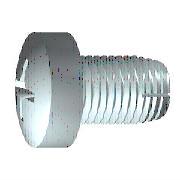
# Autodesk Inventor part: ANSI B18.6.4 - No. 4 - 40 - 1/4, CRFHTSTDTI(2)
Saved by Autodesk Inventor 2026.1 (Build 301233000, 233)
## iProperties
Created: 2025-01-21
Part Number: ANSI B18.6.4 - No. 4 - 40 - 1/4, CRFHTSTDTI(2)
Material: Steel, Mild
Description: Cross Recessed Fillister Head Tapping Screw - Type D - Type I
Document SubType Name: Modeling
Standard: ANSI B18.6.4
Designer: momen
Standard Revision: 1998
Standards Organization: ANSI
Language: en-US
Size Designation: No. 4 - 40 - 1/4
Categories: <MemberInstance><Categories><Category DisplayName="Fasteners" InternalName="e4da775c-781d-43d5-af7c-5136215cf5a6" Mnemonic="FSTN"><Category DisplayName="Bolts" InternalName="536e6df0-f778-49ac-b2f2-25c71d2aa0b2" Mnemonic="SCRW"><CategoryParameter DisplayName="Nominal Diameter Designation" InternalName="03caf894-eafd-4c09-a035-916ac084b87b" Mnemonic="nomdiadesig"/><CategoryParameter DisplayName="Nominal Length" InternalName="238ecbaf-3e6c-45dd-aa95-4068c8e0fd02" Mnemonic="nomlen"/><CategoryParameter DisplayName="Thread Designation" InternalName="586d5e89-370a-4089-914f-0110033585c7" Mnemonic="thrdesign"/><CategoryParameter DisplayName="Thread Series Designation" InternalName="87c5849c-b3a5-4c3e-9c9b-2feecef9be86" Mnemonic="thrserdsgn"/><CategoryParameter DisplayName="Nominal Diameter" InternalName="8bbe3f8e-44cf-40a9-a251-3a6edc8168d6" Mnemonic="nomdia"/><CategoryParameter DisplayName="Thread Type" InternalName="b4bbb7bc-d6aa-4c9f-a9a9-4152b9f6fe49" Mnemonic="thrtype"/><CategoryParameter DisplayName="Thread Pitch" InternalName="bb82302e-82d8-4176-8fc1-c5d7bb17d5ad" Mnemonic="pitch1"/><CategoryParameter DisplayName="Threads per Unit" InternalName="bdc6e7d2-ffd0-4d9c-a173-16b95ebb912d" Mnemonic="thrperunit1"/><CategoryParameter DisplayName="Thread Class" InternalName="ebc0d23b-2cc6-4d2a-b376-d52aae53bab6" Mnemonic="thrclss"/><Category DisplayName="Round Head" InternalName="df3578aa-538f-4805-96a8-2439eb0c3cf7" Mnemonic="RNDSCRW"><CategoryParameter DisplayName="Grip Length" InternalName="2c6ace26-543b-4217-91c4-9cdf8c3ec6f1" Mnemonic="grplen"/><CategoryParameter DisplayName="Head Height" InternalName="2d152238-84fe-49ae-94c3-3fee884c292b" Mnemonic="headh"/><CategoryParameter DisplayName="Property Class" InternalName="85496db6-1567-48ed-b0d4-aa1f03366005" Mnemonic="propclss"/><CategoryParameter DisplayName="Thread Length" InternalName="a1e5edc5-4ca7-4847-8786-65b14d35af16" Mnemonic="thrlen"/><CategoryParameter DisplayName="Shank Diameter" InternalName="c22f1a48-b8d5-43ef-ac5e-546ba91c0bd6" Mnemonic="grpdia"/><CategoryParameter DisplayName="Head Diameter" InternalName="e71ee7a1-06fd-425c-ba3b-09769885677c" Mnemonic="headdia"/><Category DisplayName="Self Tapping Screws" InternalName="33fb404f-0d7c-4133-a804-5105a5fcc9da" Mnemonic="RNDCNRGTPSCRW"/></Category></Category></Category><Category DisplayName="DataType" InternalName="23b78d0f-2648-40c6-8793-ca6db495c9e8" Mnemonic="DATATYPE"><CategoryParameter DisplayName="DisplayName" InternalName="05415f3d-3907-474b-a020-eb9d644f4cf3" Mnemonic="DISPLAYNAME"/><CategoryParameter DisplayName="Standard" InternalName="0c0a119c-1e12-4c84-803f-101930972f5e" Mnemonic="STANDARD"/><CategoryParameter DisplayName="Description" InternalName="13903e3d-64b1-4950-80da-f627842ea37f" Mnemonic="DESCRIPTION"/><CategoryParameter DisplayName="Designation" InternalName="2675968c-4ce5-49e0-a4f5-552d29089031" Mnemonic="DESIGNATION"/><CategoryParameter DisplayName="Default Row" InternalName="2af9ec52-faaa-4026-b378-f9fa4afca842" Mnemonic="DEFAULTROW"/><CategoryParameter DisplayName="Folder Name" InternalName="3f06958e-8713-4116-9be7-ed6184ecc97b" Mnemonic="FOLDERNAME"/><CategoryParameter DisplayName="Revision Guid" InternalName="45a75005-10b1-4dfc-8d6d-dfe629f0b93c" Mnemonic="REVISIONGUID"/><CategoryParameter DisplayName="FileName" InternalName="8b46a4cc-9585-4fed-90c3-899f57e09a73" Mnemonic="FILENAME"/><CategoryParameter DisplayName="StdsOrg" InternalName="8f5914e1-4693-403f-8ab5-d37768198c9d" Mnemonic="STDSORG"/><CategoryParameter DisplayName="Family Version" InternalName="914462f6-6e19-4b14-ba84-155b9680b1d0" Mnemonic="FAMILYREVISION"/><CategoryParameter DisplayName="Standard Revision" InternalName="91d5a463-65c2-4fde-b823-3b7fea5e8e17" Mnemonic="STANDARDREVISION"/><CategoryParameter DisplayName="Member Revision" InternalName="a65d44b9-392f-4f4f-857b-e4b3d54996fe" Mnemonic="MEMBERREVISION"/><CategoryParameter DisplayName="ClipFormat" InternalName="bc51e27b-3422-4e78-93ef-cec197ddf230" Mnemonic="CLIPFORMAT"/><CategoryParameter DisplayName="Manufacturer" InternalName="cd6c7a72-a28a-4e50-99a9-2c7f4e13e5ad" Mnemonic="MANUFACTURER"/><CategoryParameter DisplayName="InternalName" InternalName="cf1d0246-76d9-4b4a-8305-fa0409afb5c1" Mnemonic="INTERNALNAME"/><CategoryParameter DisplayName="IsMetric" InternalName="e2385c5b-1ea4-4823-96a8-8de651266ec3" Mnemonic="ISMETRIC"/><Category DisplayName="Part" InternalName="c0e0b642-3bcb-4cc8-9e80-f96d35c4afa4" Mnemonic="PART"><CategoryParameter DisplayName="Part Number" InternalName="016b6077-bfbe-49bd-92c9-d8d59c39c941" Mnemonic="PARTNUMBER"/><CategoryParameter DisplayName="Stock Number" InternalName="4dba7c1c-e26c-444e-836c-b08b433409a8" Mnemonic="STOCKNUMBER"/><CategoryParameter DisplayName="Material Key" InternalName="5c9a8adb-dd2b-4535-b97f-0a94a95fe41f" Mnemonic="MATERIALKEY"/><CategoryParameter DisplayName="Material" InternalName="818a152a-d3c3-49ca-80ee-df7d91421b8e" Mnemonic="MATERIAL"/></Category></Category><Category DisplayName="LegacyMap" InternalName="cd87c42b-3e48-431e-b5c0-1cbeb14dfe77" Mnemonic="LEGACYMAP"><CategoryParameter DisplayName="unique DA member ID" InternalName="0918ad47-427f-4fed-ae26-24c81c58f590" Mnemonic="DACOOKIE"/><CategoryParameter DisplayName="Merge11 ID" InternalName="0ee8fb18-e2ed-4f39-96f6-1f4b5f50aa71" Mnemonic="MERGE11"/><CategoryParameter DisplayName="unique CC member ID" InternalName="5193edd4-b2b0-4ab4-9d54-de900eee34e0" Mnemonic="CCCOOKIE"/><CategoryParameter DisplayName="Split ID" InternalName="72b5c83c-be7f-45c4-ae51-9160ea6deb26" Mnemonic="SPLIT"/><CategoryParameter DisplayName="MemberID" InternalName="8e5e0294-fc51-4c8f-b3d7-003dc5ed94f6" Mnemonic="MEMBERID"/><CategoryParameter DisplayName="CatalogName" InternalName="d99d1e27-aa94-4de2-af4c-c348882a6f4f" Mnemonic="CATALOGNAME"/><CategoryParameter DisplayName="FamilyNumber" InternalName="e705e1f4-09cb-413e-91f9-551b4188271e" Mnemonic="FAMILYNUMBER"/></Category></Categories><FamilyTemplate Id="sa0009"><FamilyTemplateParameters><FamilyTemplateParameter ObjectType="kUserParameterObject" ValueType="xs:double" Id="1" ObjectReferenceKey="KOH"/><FamilyTemplateParameter ObjectType="kUserParameterObject" ValueType="xs:double" Id="2" ObjectReferenceKey="GD2"/><FamilyTemplateParameter ObjectType="kUserParameterObject" ValueType="xs:double" Id="3" ObjectReferenceKey="KOD"/><FamilyTemplateParameter ObjectType="kUserParameterObject" ValueType="xs:double" Id="4" ObjectReferenceKey="SBR"/><FamilyTemplateParameter ObjectType="kUserParameterObject" ValueType="xs:double" Id="5" ObjectReferenceKey="KR"/><FamilyTemplateParameter ObjectType="kUserParameterObject" ValueType="xs:double" Id="6" ObjectReferenceKey="GEL"/><FamilyTemplateParameter ObjectType="kUserParameterObject" ValueType="xs:double" Id="7" ObjectReferenceKey="THREADDIA"/><FamilyTemplateParameter ObjectType="kUserParameterObject" ValueType="xs:double" Id="8" ObjectReferenceKey="TOA"/><FamilyTemplateParameter ObjectType="kUserParameterObject" ValueType="xs:double" Id="9" ObjectReferenceKey="NLG"/><FamilyTemplateParameter ObjectType="kUserParameterObject" ValueType="xs:double" Id="10" ObjectReferenceKey="STI"/><FamilyTemplateParameter ObjectType="kUserParameterObject" ValueType="xs:double" Id="11" ObjectReferenceKey="TPU"/><FamilyTemplateParameter ObjectType="kUserParameterObject" ValueType="xs:double" Id="12" ObjectReferenceKey="PTC"/><FamilyTemplateParameter ObjectType="kUserParameterObject" ValueType="xs:double" Id="13" ObjectReferenceKey="SDM"/><FamilyTemplateParameter ObjectType="kUserParameterObject" ValueType="xs:double" Id="14" ObjectReferenceKey="NND"/><FamilyTemplateParameter ObjectType="kUserParameterObject" ValueType="xs:double" Id="15" ObjectReferenceKey="SPTZ"/><FamilyTemplateParameter ObjectType="kUserParameterObject" ValueType="xs:double" Id="16" ObjectReferenceKey="GD1"/><FamilyTemplateParameter ObjectType="kPropertyObject" ValueType="xs:string" Id="100" ObjectReferenceKey="{32853F0F-3444-11d1-9E93-0060B03C1CA6}" SubObjectId="52"/><FamilyTemplateParameter ObjectType="kPropertyObject" ValueType="xs:string" Id="105" ObjectReferenceKey="{32853F0F-3444-11d1-9E93-0060B03C1CA6}" SubObjectId="5"/><FamilyTemplateParameter ObjectType="kPartComponentDefinitionObject" ValueType="xs:string" Id="110" SubObjectId="Material"/><FamilyTemplateParameter ObjectType="kThreadFeatureObject" ValueType="xs:structure" Id="300" ObjectReferenceKey="1002000010000000f2360000000000008000000000000000" SubObjectId="ThreadInfo"><FamilyTemplateParameter ObjectType="" ValueType="xs:string" Id="301" SubObjectId="ThreadDesignation"/><FamilyTemplateParameter ObjectType="" ValueType="xs:string" Id="302" SubObjectId="ThreadClass"/><FamilyTemplateParameter ObjectType="" ValueType="xs:string" Id="303" SubObjectId="ThreadType"/></FamilyTemplateParameter></FamilyTemplateParameters></FamilyTemplate><CategoryParameterMap><ParamToTemplateMap><ParamToTemplate CategoryParameter="//CategoryParameter[@InternalName='05415f3d-3907-474b-a020-eb9d644f4cf3']" ConstantValue="Cross Recessed Fillister Head Tapping Screw - Type D - Type I"/><ParamToTemplate CategoryParameter="//CategoryParameter[@InternalName='cf1d0246-76d9-4b4a-8305-fa0409afb5c1']" ConstantValue="8080ad6c-c1cb-4074-8ae5-e7158f342324"/><ParamToTemplate CategoryParameter="//CategoryParameter[@InternalName='3f06958e-8713-4116-9be7-ed6184ecc97b']" ConstantValue="ANSI B18.6.4(33)"/><ParamToTemplate CategoryParameter="//CategoryParameter[@InternalName='914462f6-6e19-4b14-ba84-155b9680b1d0']" ConstantValue="10"/><ParamToTemplate CategoryParameter="//CategoryParameter[@InternalName='bc51e27b-3422-4e78-93ef-cec197ddf230']" ConstantValue="CF_INVENTOR.STDPARTS"/><ParamToTemplate CategoryParameter="//CategoryParameter[@InternalName='e2385c5b-1ea4-4823-96a8-8de651266ec3']" ConstantValue="false"/><ParamToTemplate CategoryParameter="//CategoryParameter[@InternalName='13903e3d-64b1-4950-80da-f627842ea37f']" ConstantValue="Cross Recessed Fillister Head Tapping Screw - Type D - Type I"/><ParamToTemplate CategoryParameter="//CategoryParameter[@InternalName='8f5914e1-4693-403f-8ab5-d37768198c9d']" ConstantValue="ANSI"/><ParamToTemplate CategoryParameter="//CategoryParameter[@InternalName='0c0a119c-1e12-4c84-803f-101930972f5e']" ConstantValue="ANSI B18.6.4"/><ParamToTemplate CategoryParameter="//CategoryParameter[@InternalName='cd6c7a72-a28a-4e50-99a9-2c7f4e13e5ad']" TemplateParameter="104"/><ParamToTemplate CategoryParameter="//CategoryParameter[@InternalName='91d5a463-65c2-4fde-b823-3b7fea5e8e17']" ConstantValue="1998"/><ParamToTemplate CategoryParameter="//CategoryParameter[@InternalName='45a75005-10b1-4dfc-8d6d-dfe629f0b93c']" ConstantValue="b6542b49-97e1-4268-8fde-ea025e42451f"/><ParamToTemplate CategoryParameter="//CategoryParameter[@InternalName='2af9ec52-faaa-4026-b378-f9fa4afca842']" ConstantValue="10"/><ParamToTemplate CategoryParameter="//CategoryParameter[@InternalName='d99d1e27-aa94-4de2-af4c-c348882a6f4f']" ConstantValue="ANSI"/><ParamToTemplate CategoryParameter="//CategoryParameter[@InternalName='e705e1f4-09cb-413e-91f9-551b4188271e']" ConstantValue="949"/><ParamToTemplate CategoryParameter="//CategoryParameter[@InternalName='8b46a4cc-9585-4fed-90c3-899f57e09a73']" ConstantValue="ANSI B18.6.4 - 4-40 UNC - 0.25(3) D I"/><ParamToTemplate CategoryParameter="//CategoryParameter[@InternalName='a65d44b9-392f-4f4f-857b-e4b3d54996fe']" ConstantValue="A9A2BEB8-BFFA-4478-AFC5-B98419E7CDA5"/><ParamToTemplate CategoryParameter="//CategoryParameter[@InternalName='c22f1a48-b8d5-43ef-ac5e-546ba91c0bd6']" ConstantValue="0.112"/><ParamToTemplate CategoryParameter="//CategoryParameter[@InternalName='2c6ace26-543b-4217-91c4-9cdf8c3ec6f1']" ConstantValue="0"/><ParamToTemplate CategoryParameter="//CategoryParameter[@InternalName='ebc0d23b-2cc6-4d2a-b376-d52aae53bab6']" ConstantValue="2A"/><ParamToTemplate CategoryParameter="//CategoryParameter[@InternalName='b4bbb7bc-d6aa-4c9f-a9a9-4152b9f6fe49']" ConstantValue="ANSI Unified Screw Threads"/><ParamToTemplate CategoryParameter="//CategoryParameter[@InternalName='8e5e0294-fc51-4c8f-b3d7-003dc5ed94f6']" ConstantValue="230"/><ParamToTemplate CategoryParameter="//CategoryParameter[@InternalName='2675968c-4ce5-49e0-a4f5-552d29089031']" TemplateParameter="100"/><ParamToTemplate CategoryParameter="//CategoryParameter[@InternalName='a1e5edc5-4ca7-4847-8786-65b14d35af16']" TemplateParameter="6"/><ParamToTemplate CategoryParameter="//CategoryParameter[@InternalName='e71ee7a1-06fd-425c-ba3b-09769885677c']" TemplateParameter="3"/><ParamToTemplate CategoryParameter="//CategoryParameter[@InternalName='2d152238-84fe-49ae-94c3-3fee884c292b']" TemplateParameter="1"/><ParamToTemplate CategoryParameter="//CategoryParameter[@InternalName='818a152a-d3c3-49ca-80ee-df7d91421b8e']" TemplateParameter="110"/><ParamToTemplate CategoryParameter="//CategoryParameter[@InternalName='238ecbaf-3e6c-45dd-aa95-4068c8e0fd02']" TemplateParameter="9"/><ParamToTemplate CategoryParameter="//CategoryParameter[@InternalName='8bbe3f8e-44cf-40a9-a251-3a6edc8168d6']" TemplateParameter="14"/><ParamToTemplate CategoryParameter="//CategoryParameter[@InternalName='016b6077-bfbe-49bd-92c9-d8d59c39c941']" TemplateParameter="105"/><ParamToTemplate CategoryParameter="//CategoryParameter[@InternalName='bb82302e-82d8-4176-8fc1-c5d7bb17d5ad']" TemplateParameter="12"/><ParamToTemplate CategoryParameter="//CategoryParameter[@InternalName='586d5e89-370a-4089-914f-0110033585c7']" TemplateParameter="301"/><ParamToTemplate CategoryParameter="//CategoryParameter[@InternalName='bdc6e7d2-ffd0-4d9c-a173-16b95ebb912d']" TemplateParameter="11"/></ParamToTemplateMap></CategoryParameterMap></MemberInstance>
Density: 7.85 g/cm^3
Appearance: Semi-Polished
IsCustomPart: 0
Author: momen
Autodesk Inventor part; units mm, degrees
ref_plane "YZ Plane" through (0, 0, 0) normal (1, 0, 0) x (0, 1, 0)
sketch "Sketch1" plane through (0, 0, 0) normal (0, 0, 1) x (1, 0, 0)
  line L0 (6.35, 0) -> (6.35, 1.4224)
  line L1 (6.35, 1.4224) -> (0, 1.4224)
  arc A0 (-2.0066, 2.3241) -> (-2.7178, 0) centre (1.4352, 0) ccw
  line L2 (-2.7178, 0) -> (-2.7178, 2.3241)
  line L3 (-2.4891, 1.3592) -> (-1.3989, 0.8156)
  line L4 (-1.3989, 0.8156) -> (-0.9652, 0)
  line L5 (-4.7399, 0) -> (8.1983, 0) projected
  line L6 (0, -0.4755) -> (0, 2.8527) projected
  line L7 (-2.4891, 1.3592) -> (-2.7178, 1.4732) construction
  line L8 (-2.0066, 2.3241) -> (-2.7178, 2.3241)
  line L9 (-2.0066, 2.3241) -> (0, 2.3241)
  dimension "d0" = 1.7526
  dimension "d10" = 2.7178
  dimension "d11" = 6.35
  dimension "d12" = 2.8448
  dimension "d13" = 2.9464
  dimension "d14" = 4.6482
  dimension "d15" = 26.5
  dimension "d16" = 62
  dimension "d17" = 0.7112
  constraints: 16 end point, 8 point on line, 4 point on circle, 2 collinear, 1 centre point, 1 tangent
  measures "d0" distance from line of L4.end L2
  measures "d10" distance between parallel lines of L6 L2
  measures "d11" distance between parallel lines of L6 L0
  measures "d12" diameter of L1 L5
  measures "d13" diameter of L7.end L5
  measures "d14" diameter of L9 L5
  measures "d15" angle of L5 L3
  measures "d16" angle of L5 L4
  measures "d17" distance from line of L2 L8.start
revolve "Body" add sketch "Sketch1" angle 360 about axis through (-10, 0, 0) along (1, 0, 0) contours L5 L6 L1 L0 | L5 L4 L3 A0 L9 L6
ref_plane "IDS_WORKPLANE{1}" through (-2.7178, 0, 0) normal (1, 0, 0) x (0, 1, 0)
sketch "Sketch2" plane through (-2.7178, 0, 0) normal (1, 0, 0) x (0, 1, 0)
  circle A0 centre (0, 0) radius 2.3241 projected
  line L0 (-4.1281, 0) -> (8.4996, 0) projected
  line L1 (0, -4.1281) -> (0, 8.4996) projected
  line L2 (0, 1.4732) -> (0, 0) construction
  line L3 (0, 0) -> (1.4732, 0) construction
  arc A1 (0.4911, 0) -> (0, 0.4911) centre (0, 0) ccw construction
  line L4 (0, 0) -> (6.6957, 6.6957) construction
  line L5 (0.2413, 1.4533) -> (0.2077, 0.7067)
  line L6 (1.4533, 0.2413) -> (0.7067, 0.2077)
  arc A2 (1.4732, 0) -> (1.4533, 0.2413) centre (0, 0) ccw
  arc A3 (0.2413, 1.4533) -> (0, 1.4732) centre (0, 0) ccw
  arc A4 (1.4533, 0.2413) -> (0.2413, 1.4533) centre (0, 0) ccw
  arc A5 (1.4533, -0.2413) -> (1.4732, 0) centre (0, 0) ccw
  arc A6 (0, -1.4732) -> (0.2413, -1.4533) centre (0, 0) ccw
  arc A7 (0.2413, -1.4533) -> (1.4533, -0.2413) centre (0, 0) ccw
  arc A8 (-1.4533, 0.2413) -> (-1.4732, 0) centre (0, 0) ccw
  arc A9 (0, 1.4732) -> (-0.2413, 1.4533) centre (0, 0) ccw
  arc A10 (-0.2413, 1.4533) -> (-1.4533, 0.2413) centre (0, 0) ccw
  arc A11 (-0.2413, -1.4533) -> (0, -1.4732) centre (0, 0) ccw
  arc A12 (-1.4533, -0.2413) -> (-0.2413, -1.4533) centre (0, 0) ccw
  arc A13 (-1.4732, 0) -> (-1.4533, -0.2413) centre (0, 0) ccw
  arc A14 (0.7366, 0) -> (0, 0.7366) centre (0, 0) ccw construction
  arc A15 (0.2077, 0.7067) -> (0.7067, 0.2077) centre (0.6852, 0.6852) ccw
  line L7 (0.2413, -1.4533) -> (0.2077, -0.7067)
  line L8 (1.4533, -0.2413) -> (0.7067, -0.2077)
  arc A16 (0.7067, -0.2077) -> (0.2077, -0.7067) centre (0.6852, -0.6852) ccw
  line L9 (-0.2413, 1.4533) -> (-0.2077, 0.7067)
  line L10 (-1.4533, 0.2413) -> (-0.7067, 0.2077)
  arc A17 (-0.7067, 0.2077) -> (-0.2077, 0.7067) centre (-0.6852, 0.6852) ccw
  line L11 (-0.2413, -1.4533) -> (-0.2077, -0.7067)
  arc A18 (-0.2077, -0.7067) -> (-0.7067, -0.2077) centre (-0.6852, -0.6852) ccw
  line L12 (-1.4533, -0.2413) -> (-0.7067, -0.2077)
  dimension "d2" = 45
  dimension "d3" = 0.9821
  dimension "d4" = 2.9464
  dimension "d5" = 0.2413
  dimension "d7" = 1.4732
  constraints: 38 point on circle, 22 end point, 19 symmetric about line, 18 centre point, 4 coincident, 3 collinear, 3 tangent, 2 point on line, 1 midpoint, 1 perpendicular, 19 other
  measures "d2" angle of L4 L3
  measures "d3" diameter of A1
  measures "d4" diameter of A4
  measures "d5" distance from line of L5.start L2
  measures "d7" diameter of A14
extrude "Slot" add sketch "Sketch2" along normal up to next draft 0.5 contours L6 A15 L5 A4 | A7 L7 A16 L8 | L9 A17 L10 A10 | A12 L12 A18 L11
revolve "Cut" cut sketch "Sketch1" angle 360 about axis through (-10, 0, 0) along (1, 0, 0) contours L2 L8 A0
fillet "Fillet1" radius 0.0965 5 edges at (-2.4891, 0, -1.3592) (-2.4891, 1.3541, 0.1175) (-2.4891, 1.3541, -0.1175) (-2.4891, 0, 1.3592) (-2.4891, -1.3592, 0)
thread "Thread" size "4-40 UNC" class "2A" standard "ANSI Unified Screw Threads" length 6.35
chamfer "Chamfer1" distance 0.3175 distance2 2.2352 1 edges at (6.35, -1.4224, 0) measured on face at (6.35, 0.2331, 0.9781)
ref_plane "Work Plane3" through (2.3812, 0, 0) normal (0, 1, 0) x (1, 0, 0)
equation "\"d3\" = 0.333333 * SDM"
equation "\"d4\" = SDM"
equation "\"d5\" = 0.5 * SBR"
equation "\"d7\" = 0.5 * SDM"
equation "\"d0\" = STI"
equation "\"d10\" = KOH"
equation "\"d11\" = NLG"
equation "\"d12\" = NND"
equation "\"d13\" = SDM"
equation "\"d14\" = KOD"
equation "\"d17\" = KR"
equation "\"d19\" = 0.2 * SBR"
equation "\"d20\" = GEL"
equation "\"d22\" = -0.5 * GD2 + 0.5 * NND"
equation "\"d23\" = SPTZ"
equation "\"NND\" = 2.8448"
equation "\"NLG\" = 6.35"
equation "\"GEL\" = 6.35"
equation "\"KOD\" = 4.6482"
equation "\"KOH\" = 2.7178"
equation "\"SDM\" = 2.9464"
equation "\"STI\" = 1.7526"
equation "\"SBR\" = 0.4826"
equation "\"d1\" = -KOH"
equation "\"KR\" = 0.7112"
equation "\"SPTZ\" = 2.2352"
equation "\"GD2\" = 2.2098"
equation "\"THREADDIA\" = 2.8448"
equation "\"TOA\" = 30deg"
equation "\"GD1\" = 2.2098"
body "Solid1"
